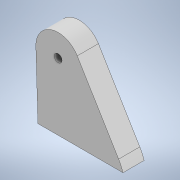
# Autodesk Inventor part: heaript
Saved by Autodesk Inventor 2020 (Build 240168000, 168)
## iProperties
Created: 2022-10-17
Part Number: heaript
Material: Типовые
Document SubType Name: Modeling
Designer: zigma
Density: 1 g/cm^3
Appearance: По умолчанию
Author: zigma
Autodesk Inventor part; units mm, degrees
ref_plane "YZ Plane" through (0, 0, 0) normal (1, 0, 0) x (0, 1, 0)
ref_plane "XZ Plane" through (0, 0, 0) normal (0, 1, 0) x (-1, 0, 0)
ref_plane "XY Plane" through (0, 0, 0) normal (0, 0, 1) x (1, 0, 0)
sketch "Эскиз1" plane through (0, 0, 0) normal (0, 0, 1) x (1, 0, 0)
  arc A0 (19.0788, 6) -> (17.1347, 10.3152) centre (0, 0) ccw
  line L0 (-19.0788, 6) -> (19.0788, 6)
  circle A1 centre (-10, 36) radius 1.75
  circle A2 centre (-10, 36) radius 10
  line L1 (-19.9952, 35.6915) -> (-19.0788, 6)
  line L2 (-1.4327, 41.1576) -> (17.1347, 10.3152)
  dimension "d0" = 40
  dimension "d1" = 6
  dimension "d2" = 3.5
  dimension "d3" = 20
  dimension "d4" = 30
  dimension "d5" = 10
  constraints: 6 end point, 4 point on circle, 3 centre point, 3 tangent, 2 coincident, 1 horizontal
  measures "d0" diameter of A0
  measures "d1" distance from line of point (0, 0) L0
  measures "d2" diameter of A1
  measures "d3" diameter of A2
  measures "d4" distance from line of L0 A2.centre
  measures "d5" horizontal distance of point (0, 0) A2.centre
extrude "Выдавливание1" add sketch "Эскиз1" along normal blind 9.5
